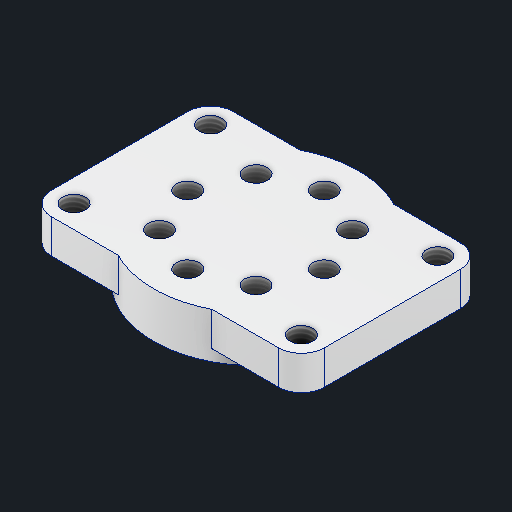
# Autodesk Inventor part: ArmBearingClampingPlate2
Saved by Autodesk Inventor 2025 (Build 290162000, 162)
## iProperties
Created: 2024-05-20
Part Number: ArmBearingClampingPlate2
Material: Aluminum 6061
Document SubType Name: Modeling
Designer: avsar
Density: 2.7 g/cm^3
Appearance: Aluminum - Flat
Author: avsar
Autodesk Inventor part; units mm, degrees
ref_plane "YZ Plane" through (0, 0, 0) normal (1, 0, 0) x (0, 1, 0)
ref_plane "XZ Plane" through (0, 0, 0) normal (0, 1, 0) x (-1, 0, 0)
ref_plane "XY Plane" through (0, 0, 0) normal (0, 0, 1) x (1, 0, 0)
sketch "Sketch1" plane through (0, 0, 0) normal (0, 1, 0) x (-1, 0, 0)
  circle A0 centre (0, 0) radius 18
  circle A1 centre (0, -12) radius 2
  circle A2 centre (8.4853, -8.4853) radius 2
  circle A3 centre (12, 0) radius 2
  circle A4 centre (8.4853, 8.4853) radius 2
  circle A5 centre (0, 12) radius 2
  circle A6 centre (-8.4853, 8.4853) radius 2
  circle A7 centre (-12, 0) radius 2
  circle A8 centre (-8.4853, -8.4853) radius 2
  dimension "d0" = 36
  dimension "d1" = 4
  dimension "d2" = 12
  dimension "d5" = 360
  constraints: 9 centre point, 1 coincident, 1 vertical alignment, 17 other
  measures "d0" diameter of A0
  measures "d1" diameter of A1
  measures "d2" distance of point (0, 0) A1.centre
extrude "Extrusion1" add sketch "Sketch1" along normal blind 8
thread "Thread1" size "M4x0.7" class "6H" standard "ANSI Metric M Profile" full length
thread "Thread2" size "M4x0.7" class "6H" standard "ANSI Metric M Profile" full length
thread "Thread3" size "M4x0.7" class "6H" standard "ANSI Metric M Profile" full length
thread "Thread4" size "M4x0.7" class "6H" standard "ANSI Metric M Profile" full length
thread "Thread5" size "M4x0.7" class "6H" standard "ANSI Metric M Profile" full length
thread "Thread6" size "M4x0.7" class "6H" standard "ANSI Metric M Profile" full length
thread "Thread7" size "M4x0.7" class "6H" standard "ANSI Metric M Profile" full length
thread "Thread8" size "M4x0.7" class "6H" standard "ANSI Metric M Profile" full length
sketch "Sketch2" plane through (0, 8, 0) normal (0, 1, 0) x (1, 0, 0)
  line L0 (-24, -16) -> (24, -16)
  line L1 (24, -16) -> (24, 16)
  line L2 (24, 16) -> (-24, 16)
  line L3 (-24, 16) -> (-24, -16)
  line L4 (-24, -16) -> (24, 16) construction
  line L5 (24, -16) -> (-24, 16) construction
  circle A0 centre (-20, 12) radius 2
  line L6 (0, 0) -> (0, -16) construction
  line L7 (0, 0) -> (24, 0) construction
  circle A1 centre (0, 0) radius 18 projected
  circle A2 centre (8.4853, 8.4853) radius 2 projected
  circle A3 centre (12, 0) radius 2 projected
  circle A4 centre (8.4853, -8.4853) radius 2 projected
  circle A5 centre (0, -12) radius 2 projected
  circle A6 centre (-8.4853, -8.4853) radius 2 projected
  circle A7 centre (-12, 0) radius 2 projected
  circle A8 centre (-8.4853, 8.4853) radius 2 projected
  circle A9 centre (0, 12) radius 2 projected
  circle A10 centre (20, 12) radius 2
  circle A11 centre (-20, -12) radius 2
  circle A12 centre (20, -12) radius 2
  point P0 (8.2462, 16)
  point P1 (8.2462, -16)
  point P2 (-8.2462, -16)
  point P3 (-8.2462, 16)
  dimension "d25" = 48
  dimension "d26" = 32
  dimension "d27" = 4
  dimension "d28" = 20
  dimension "d29" = 12
  constraints: 16 end point, 4 centre point, 4 midpoint, 3 symmetric about line, 2 parallel, 1 horizontal, 1 perpendicular, 3 other
  measures "d25" distance of L2.end L1.end
  measures "d26" distance of L1.end L0.end
  measures "d27" diameter of A0
  measures "d28" horizontal distance of A0.centre L6.start
  measures "d29" vertical distance of L6.start A0.centre
extrude "Extrusion2" add sketch "Sketch2" against normal blind 6 contours L3 L2 A1 L0 | A1 L2 L1 L0
fillet "Fillet1" radius 4 4 edges at (-24, 5, 16) (24, 5, 16) (24, 5, -16) (-24, 5, -16)
thread "Thread9" size "M4.5x0.75" class "6H" standard "ANSI Metric M Profile" full length
thread "Thread10" size "M4.5x0.75" class "6H" standard "ANSI Metric M Profile" full length
thread "Thread11" size "M4.5x0.75" class "6H" standard "ANSI Metric M Profile" full length
thread "Thread12" size "M4.5x0.75" class "6H" standard "ANSI Metric M Profile" full length
body "Solid1"
